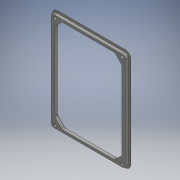
# Autodesk Inventor part: SolarPanel_CoilForm
Saved by Autodesk Inventor 2018 (Build 220112000, 112)
## iProperties
Created: 2018-05-13
Part Number: SolarPanel_CoilForm
Material: ABS Plastic
Document SubType Name: Modeling
Designer: Bradley
Density: 1.06 g/cm^3
Appearance: Smooth - Medium Gray
Author: Bradley
Autodesk Inventor part; units mm, degrees
ref_plane "YZ Plane" through (0, 0, 0) normal (1, 0, 0) x (0, 1, 0)
ref_plane "XZ Plane" through (0, 0, 0) normal (0, 1, 0) x (-1, 0, 0)
ref_plane "XY Plane" through (0, 0, 0) normal (0, 0, 1) x (1, 0, 0)
sketch "Sketch1" plane through (0, 0, 0) normal (0, 1, 0) x (-1, 0, 0)
  line L0 (32.5, 45) -> (-32.5, 45) construction
  line L1 (-32.5, 45) -> (-32.5, -45) construction
  line L2 (-32.5, -45) -> (32.5, -45) construction
  line L3 (32.5, -45) -> (32.5, 45) construction
  line L4 (33, 49.5) -> (-33, 49.5)
  line L5 (-38, 44.5) -> (-38, -44.5)
  line L6 (-33, -49.5) -> (33, -49.5)
  line L7 (38, -44.5) -> (38, 44.5)
  arc A0 (38, 44.5) -> (33, 49.5) centre (33, 44.5) ccw
  arc A1 (-33, 49.5) -> (-38, 44.5) centre (-33, 44.5) ccw
  arc A2 (-38, -44.5) -> (-33, -49.5) centre (-33, -44.5) ccw
  arc A3 (33, -49.5) -> (38, -44.5) centre (33, -44.5) ccw
  line L8 (-33, 47.5) -> (33, 47.5)
  arc A4 (36, 44.5) -> (33, 47.5) centre (33, 44.5) ccw
  line L9 (36, 44.5) -> (36, -44.5)
  arc A5 (33, -47.5) -> (36, -44.5) centre (33, -44.5) ccw
  line L10 (33, -47.5) -> (-33, -47.5)
  arc A6 (-36, -44.5) -> (-33, -47.5) centre (-33, -44.5) ccw
  line L11 (-36, -44.5) -> (-36, 44.5)
  arc A7 (-33, 47.5) -> (-36, 44.5) centre (-33, 44.5) ccw
  circle A8 centre (32.5, 45) radius 1.65
  circle A9 centre (32.5, -45) radius 1.65
  circle A10 centre (-32.5, -45) radius 1.65
  circle A11 centre (-32.5, 45) radius 1.65
  line L12 (32.5, 38) -> (25.5, 45)
  line L13 (25.5, 45) -> (-25.5, 45)
  line L14 (-25.5, 45) -> (-32.5, 38)
  line L15 (-32.5, 38) -> (-32.5, -38)
  line L16 (-32.5, -38) -> (-25.5, -45)
  line L17 (-25.5, -45) -> (25.5, -45)
  line L18 (25.5, -45) -> (32.5, -38)
  line L19 (32.5, -38) -> (32.5, 38)
  point P0 (0, 0)
  point P1 (32.5, 0)
  point P2 (38, 49.5)
  point P3 (-38, 49.5)
  point P4 (38, -49.5)
  point P5 (-38, 0)
  point P6 (0, 49.5)
  point P7 (0, 45)
  dimension "d0" = 76
  dimension "d1" = 99
  dimension "d2" = 5
  dimension "d3" = 2
  dimension "d4" = 3.3
  dimension "d5" = 0.85
  dimension "d6" = 1.85
  dimension "d7" = 65
  dimension "d8" = 90
  dimension "d9" = 7
  dimension "d10" = 4.9497
  constraints: 40 end point, 16 point on circle, 14 point on line, 12 centre point, 9 perpendicular, 8 tangent, 6 equal radius, 6 parallel, 5 midpoint, 4 coincident, 2 horizontal, 2 horizontal alignment, 2 vertical alignment, 7 other
  measures "d0" distance of point (38, 49.5) point (-38, 49.5)
  measures "d1" distance of point (38, -49.5) point (38, 49.5)
  measures "d2" radius of A0
  measures "d3" distance between parallel lines of L9 L7
  measures "d4" diameter of A8
  measures "d5" distance edge to line of A8 L8
  measures "d6" distance edge to line of A8 L9
  measures "d7" distance of L0.start L0.end
  measures "d8" distance of L2.end L0.start
  measures "d9" horizontal distance of L12.start L12.end
  measures "d10" distance from line of L0.start L12
extrude "Extrusion1" add sketch "Sketch1" along normal mid plane 3.25 contours A0 L7 A3 L6 A2 L5 A1 L4 | L8 A4 L9 A5 L10 A6 L11 A7
fillet "Fillet1" radius 2 8 edges at (-32.5, 0, -38) (-25.5, 0, -45) (25.5, 0, -45) (32.5, 0, -38) (32.5, 0, 38) (25.5, 0, 45) (-32.5, 0, 38) (-25.5, 0, 45)
sketch "Sketch2" plane through (0, -1.625, 0) normal (0, -1, 0) x (1, 0, 0)
  line L0 (-36, 44.5) -> (-36, -44.5) projected
  arc A0 (-33, 47.5) -> (-36, 44.5) centre (-33, 44.5) ccw projected
  line L1 (33, 47.5) -> (-33, 47.5) projected
  arc A1 (36, 44.5) -> (33, 47.5) centre (33, 44.5) ccw projected
  line L2 (-32.5, 37.1716) -> (-32.5, -37.1716) projected
  arc A2 (-32.5, -37.1716) -> (-31.9142, -38.5858) centre (-30.5, -37.1716) ccw projected
  line L3 (-31.9142, -38.5858) -> (-26.0858, -44.4142) projected
  arc A3 (-26.0858, -44.4142) -> (-24.6716, -45) centre (-24.6716, -43) ccw projected
  line L4 (-24.6716, -45) -> (24.6716, -45) projected
  arc A4 (24.6716, -45) -> (26.0858, -44.4142) centre (24.6716, -43) ccw projected
  line L5 (26.0858, -44.4142) -> (31.9142, -38.5858) projected
  arc A5 (31.9142, -38.5858) -> (32.5, -37.1716) centre (30.5, -37.1716) ccw projected
  line L6 (32.5, -37.1716) -> (32.5, 37.1716) projected
  arc A6 (32.5, 37.1716) -> (31.9142, 38.5858) centre (30.5, 37.1716) ccw projected
  line L7 (31.9142, 38.5858) -> (26.0858, 44.4142) projected
  arc A7 (26.0858, 44.4142) -> (24.6716, 45) centre (24.6716, 43) ccw projected
  line L8 (24.6716, 45) -> (-24.6716, 45) projected
  arc A8 (-24.6716, 45) -> (-26.0858, 44.4142) centre (-24.6716, 43) ccw projected
  line L9 (-26.0858, 44.4142) -> (-31.9142, 38.5858) projected
  arc A9 (-31.9142, 38.5858) -> (-32.5, 37.1716) centre (-30.5, 37.1716) ccw projected
  circle A10 centre (32.5, 45) radius 1.65 projected
  circle A11 centre (32.5, -45) radius 1.65 projected
  circle A12 centre (-32.5, -45) radius 1.65 projected
  circle A13 centre (-32.5, 45) radius 1.65 projected
  line L10 (-33, 49.5) -> (33, 49.5) projected
  arc A14 (38, 44.5) -> (33, 49.5) centre (33, 44.5) ccw projected
  line L11 (38, 44.5) -> (38, -44.5) projected
  arc A15 (33, -49.5) -> (38, -44.5) centre (33, -44.5) ccw projected
  line L12 (33, -49.5) -> (-33, -49.5) projected
  arc A16 (-38, -44.5) -> (-33, -49.5) centre (-33, -44.5) ccw projected
  line L13 (-38, -44.5) -> (-38, 44.5) projected
  arc A17 (-33, 49.5) -> (-38, 44.5) centre (-33, 44.5) ccw projected
  line L14 (36, -44.5) -> (36, 44.5) projected
  arc A18 (33, -47.5) -> (36, -44.5) centre (33, -44.5) ccw projected
  line L15 (-33, -47.5) -> (33, -47.5) projected
  arc A19 (-36, -44.5) -> (-33, -47.5) centre (-33, -44.5) ccw projected
  point P0 (0, 0)
extrude "Extrusion3" cut sketch "Sketch2" against normal blind 2.75 contours L10 A14 L11 A15 L12 A16 L13 A17
chamfer "Chamfer1" distance 0.5 angle 45 16 edges at (-29, 1.625, 41.5) (-32.3478, 1.625, 37.9369) (-32.5, 1.625, 0) (-32.3478, 1.625, -37.9369) (-29, 1.625, -41.5) (-25.4369, 1.625, -44.8478) (0, 1.625, -45) (25.4369, 1.625, -44.8478) (29, 1.625, -41.5) (32.3478, 1.625, -37.9369) (32.5, 1.625, 0) (32.3478, 1.625, 37.9369) (29, 1.625, 41.5) (25.4369, 1.625, 44.8478) (0, 1.625, 45) (-25.4369, 1.625, 44.8478)
body "Solid1"
